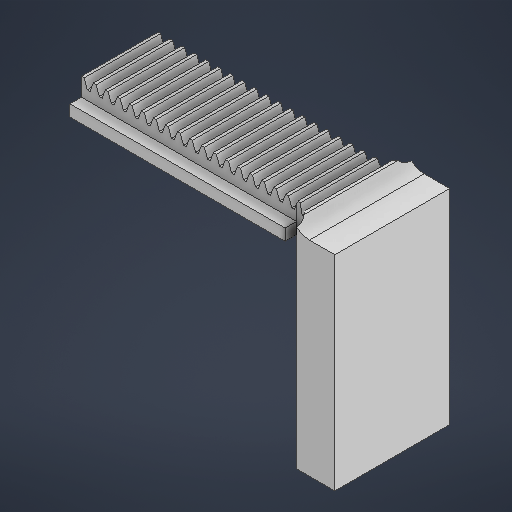
# Autodesk Inventor part: cremallera 4
Saved by Autodesk Inventor 2025.3 (Build 293356000, 356)
## iProperties
Created: 2025-10-14
Part Number: cremallera 4
Material: Genérico
Document SubType Name: Modeling
Designer: Jonathan Galarza
Density: 1 g/cm^3
Appearance: Valor por defecto
Author: Jonathan Galarza
Autodesk Inventor part; units mm, degrees
ref_plane "YZ Plane" through (0, 0, 0) normal (1, 0, 0) x (0, 1, 0)
ref_plane "XZ Plane" through (0, 0, 0) normal (0, 1, 0) x (-1, 0, 0)
ref_plane "XY Plane" through (0, 0, 0) normal (0, 0, 1) x (1, 0, 0)
sketch "Boceto1" plane through (0, 0, 0) normal (0, 0, 1) x (1, 0, 0)
  line L0 (-18.1967, 3.5798) -> (-17.4337, 3.5798)
  line L1 (-17.4337, 3.5798) -> (-16.6075, 1.3098)
  line L2 (-17.4337, 3.5798) -> (-14.4337, 3.5798) construction
  line L3 (-17.0697, 2.5798) -> (-18.5607, 2.5798) construction
  line L4 (-17.8152, 2.5798) -> (-17.8152, 2.7741) construction
  line L5 (-18.1967, 3.5798) -> (-19.023, 1.3098)
  line L6 (-15.0557, 3.5798) -> (-14.2927, 3.5798)
  line L7 (-14.2927, 3.5798) -> (-13.4665, 1.3098)
  line L8 (-13.9287, 2.5798) -> (-15.4197, 2.5798) construction
  line L9 (-14.6742, 2.5798) -> (-14.6742, 2.7741) construction
  line L10 (-15.0557, 3.5798) -> (-15.882, 1.3098)
  line L11 (-11.9147, 3.5798) -> (-11.1517, 3.5798)
  line L12 (-11.1517, 3.5798) -> (-10.3255, 1.3098)
  line L13 (-10.7877, 2.5798) -> (-12.2787, 2.5798) construction
  line L14 (-11.5332, 2.5798) -> (-11.5332, 2.7741) construction
  line L15 (-11.9147, 3.5798) -> (-12.741, 1.3098)
  line L16 (-8.7737, 3.5798) -> (-8.0107, 3.5798)
  line L17 (-8.0107, 3.5798) -> (-7.1845, 1.3098)
  line L18 (-7.6467, 2.5798) -> (-9.1377, 2.5798) construction
  line L19 (-8.3922, 2.5798) -> (-8.3922, 2.7741) construction
  line L20 (-8.7737, 3.5798) -> (-9.6, 1.3098)
  line L21 (-5.6327, 3.5798) -> (-4.8697, 3.5798)
  line L22 (-4.8697, 3.5798) -> (-4.0435, 1.3098)
  line L23 (-4.5057, 2.5798) -> (-5.9967, 2.5798) construction
  line L24 (-5.2512, 2.5798) -> (-5.2512, 2.7741) construction
  line L25 (-5.6327, 3.5798) -> (-6.459, 1.3098)
  line L26 (-2.4917, 3.5798) -> (-1.7287, 3.5798)
  line L27 (-1.7287, 3.5798) -> (-0.9025, 1.3098)
  line L28 (-1.3647, 2.5798) -> (-2.8557, 2.5798) construction
  line L29 (-2.1102, 2.5798) -> (-2.1102, 2.7741) construction
  line L30 (-2.4917, 3.5798) -> (-3.318, 1.3098)
  line L31 (0.6493, 3.5798) -> (1.4123, 3.5798)
  line L32 (1.4123, 3.5798) -> (2.2385, 1.3098)
  line L33 (1.7763, 2.5798) -> (0.2853, 2.5798) construction
  line L34 (1.0308, 2.5798) -> (1.0308, 2.7741) construction
  line L35 (0.6493, 3.5798) -> (-0.177, 1.3098)
  line L36 (3.7903, 3.5798) -> (4.5533, 3.5798)
  line L37 (4.5533, 3.5798) -> (5.3795, 1.3098)
  line L38 (4.9173, 2.5798) -> (3.4263, 2.5798) construction
  line L39 (4.1718, 2.5798) -> (4.1718, 2.7741) construction
  line L40 (3.7903, 3.5798) -> (2.964, 1.3098)
  line L41 (6.9313, 3.5798) -> (7.6943, 3.5798)
  line L42 (7.6943, 3.5798) -> (8.5205, 1.3098)
  line L43 (8.0583, 2.5798) -> (6.5673, 2.5798) construction
  line L44 (7.3128, 2.5798) -> (7.3128, 2.7741) construction
  line L45 (6.9313, 3.5798) -> (6.105, 1.3098)
  line L46 (10.0723, 3.5798) -> (10.8353, 3.5798)
  line L47 (10.8353, 3.5798) -> (11.6615, 1.3098)
  line L48 (11.1993, 2.5798) -> (9.7083, 2.5798) construction
  line L49 (10.4538, 2.5798) -> (10.4538, 2.7741) construction
  line L50 (10.0723, 3.5798) -> (9.246, 1.3098)
  line L51 (13.2133, 3.5798) -> (13.9763, 3.5798)
  line L52 (13.9763, 3.5798) -> (14.8025, 1.3098)
  line L53 (14.3403, 2.5798) -> (12.8493, 2.5798) construction
  line L54 (13.5948, 2.5798) -> (13.5948, 2.7741) construction
  line L55 (13.2133, 3.5798) -> (12.387, 1.3098)
  line L56 (16.3543, 3.5798) -> (17.1173, 3.5798)
  line L57 (17.1173, 3.5798) -> (17.9435, 1.3098)
  line L58 (17.4813, 2.5798) -> (15.9903, 2.5798) construction
  line L59 (16.7358, 2.5798) -> (16.7358, 2.7741) construction
  line L60 (16.3543, 3.5798) -> (15.528, 1.3098)
  line L61 (19.4953, 3.5798) -> (20.2583, 3.5798)
  line L62 (20.2583, 3.5798) -> (21.0845, 1.3098)
  line L63 (20.6223, 2.5798) -> (19.1313, 2.5798) construction
  line L64 (19.8768, 2.5798) -> (19.8768, 2.7741) construction
  line L65 (19.4953, 3.5798) -> (18.669, 1.3098)
  line L66 (22.6363, 3.5798) -> (23.3993, 3.5798)
  line L67 (23.3993, 3.5798) -> (24.2255, 1.3098)
  line L68 (23.7633, 2.5798) -> (22.2723, 2.5798) construction
  line L69 (23.0178, 2.5798) -> (23.0178, 2.7741) construction
  line L70 (22.6363, 3.5798) -> (21.81, 1.3098)
  line L71 (25.7773, 3.5798) -> (26.5403, 3.5798)
  line L72 (26.5403, 3.5798) -> (27.3665, 1.3098)
  line L73 (26.9043, 2.5798) -> (25.4133, 2.5798) construction
  line L74 (26.1588, 2.5798) -> (26.1588, 2.7741) construction
  line L75 (25.7773, 3.5798) -> (24.951, 1.3098)
  line L76 (28.9183, 3.5798) -> (29.6813, 3.5798)
  line L77 (29.6813, 3.5798) -> (30.5075, 1.3098)
  line L78 (30.0453, 2.5798) -> (28.5543, 2.5798) construction
  line L79 (29.2998, 2.5798) -> (29.2998, 2.7741) construction
  line L80 (28.9183, 3.5798) -> (28.092, 1.3098)
  line L81 (32.0593, 3.5798) -> (32.8223, 3.5798)
  line L82 (32.8223, 3.5798) -> (33.6485, 1.3098)
  line L83 (33.1863, 2.5798) -> (31.6953, 2.5798) construction
  line L84 (32.4408, 2.5798) -> (32.4408, 2.7741) construction
  line L85 (32.0593, 3.5798) -> (31.233, 1.3098)
  line L86 (35.2003, 3.5798) -> (35.9633, 3.5798)
  line L87 (35.9633, 3.5798) -> (36.7895, 1.3098)
  line L88 (36.3273, 2.5798) -> (34.8363, 2.5798) construction
  line L89 (35.5818, 2.5798) -> (35.5818, 2.7741) construction
  line L90 (35.2003, 3.5798) -> (34.374, 1.3098)
  line L91 (38.3413, 3.5798) -> (39.1043, 3.5798)
  line L92 (39.1043, 3.5798) -> (39.9305, 1.3098)
  line L93 (39.4683, 2.5798) -> (37.9773, 2.5798) construction
  line L94 (38.7228, 2.5798) -> (38.7228, 2.7741) construction
  line L95 (38.3413, 3.5798) -> (37.515, 1.3098)
  line L96 (41.4823, 3.5798) -> (42.2453, 3.5798)
  line L97 (42.2453, 3.5798) -> (43.0715, 1.3098)
  line L98 (42.6093, 2.5798) -> (41.1183, 2.5798) construction
  line L99 (41.8638, 2.5798) -> (41.8638, 2.7741) construction
  line L100 (41.4823, 3.5798) -> (40.656, 1.3098)
  line L101 (44.6233, 3.5798) -> (45.3863, 3.5798)
  line L102 (45.3863, 3.5798) -> (46.2125, 1.3098)
  line L103 (45.7503, 2.5798) -> (44.2593, 2.5798) construction
  line L104 (45.0048, 2.5798) -> (45.0048, 2.7741) construction
  line L105 (44.6233, 3.5798) -> (43.797, 1.3098)
  line L106 (47.7643, 3.5798) -> (48.5273, 3.5798)
  line L107 (48.5273, 3.5798) -> (49.3535, 1.3098)
  line L108 (48.8913, 2.5798) -> (47.4003, 2.5798) construction
  line L109 (48.1458, 2.5798) -> (48.1458, 2.7741) construction
  line L110 (47.7643, 3.5798) -> (46.938, 1.3098)
  line L111 (50.9053, 3.5798) -> (51.6683, 3.5798)
  line L112 (51.6683, 3.5798) -> (52.4945, 1.3098)
  line L113 (52.0323, 2.5798) -> (50.5413, 2.5798) construction
  line L114 (51.2868, 2.5798) -> (51.2868, 2.7741) construction
  line L115 (50.9053, 3.5798) -> (50.079, 1.3098)
  line L116 (54.0463, 3.5798) -> (54.8093, 3.5798)
  line L117 (54.8093, 3.5798) -> (55.6355, 1.3098)
  line L118 (55.1733, 2.5798) -> (53.6823, 2.5798) construction
  line L119 (54.4278, 2.5798) -> (54.4278, 2.7741) construction
  line L120 (54.0463, 3.5798) -> (53.22, 1.3098)
  line L121 (57.1873, 3.5798) -> (57.9503, 3.5798)
  line L122 (57.9503, 3.5798) -> (58.7765, 1.3098)
  line L123 (58.3143, 2.5798) -> (56.8233, 2.5798) construction
  line L124 (57.5688, 2.5798) -> (57.5688, 2.7741) construction
  line L125 (57.1873, 3.5798) -> (56.361, 1.3098)
  line L126 (60.3283, 3.5798) -> (61.0913, 3.5798)
  line L127 (61.0913, 3.5798) -> (61.9175, 1.3098)
  line L128 (61.4553, 2.5798) -> (59.9643, 2.5798) construction
  line L129 (60.7098, 2.5798) -> (60.7098, 2.7741) construction
  line L130 (60.3283, 3.5798) -> (59.502, 1.3098)
  line L131 (63.4693, 3.5798) -> (64.2323, 3.5798)
  line L132 (64.2323, 3.5798) -> (65.0585, 1.3098)
  line L133 (64.5963, 2.5798) -> (63.1053, 2.5798) construction
  line L134 (63.8508, 2.5798) -> (63.8508, 2.7741) construction
  line L135 (63.4693, 3.5798) -> (62.643, 1.3098)
  line L136 (66.6103, 3.5798) -> (67.3733, 3.5798)
  line L137 (67.3733, 3.5798) -> (68.1995, 1.3098)
  line L138 (67.7373, 2.5798) -> (66.2463, 2.5798) construction
  line L139 (66.9918, 2.5798) -> (66.9918, 2.7741) construction
  line L140 (66.6103, 3.5798) -> (65.784, 1.3098)
  line L141 (69.7513, 3.5798) -> (70.5143, 3.5798)
  line L142 (70.5143, 3.5798) -> (71.3405, 1.3098)
  line L143 (70.8783, 2.5798) -> (69.3873, 2.5798) construction
  line L144 (70.1328, 2.5798) -> (70.1328, 2.7741) construction
  line L145 (69.7513, 3.5798) -> (68.925, 1.3098)
  line L146 (72.8923, 3.5798) -> (73.6553, 3.5798)
  line L147 (73.6553, 3.5798) -> (74.4815, 1.3098)
  line L148 (74.0193, 2.5798) -> (72.5283, 2.5798) construction
  line L149 (73.2738, 2.5798) -> (73.2738, 2.7741) construction
  line L150 (72.8923, 3.5798) -> (72.066, 1.3098)
  line L151 (-19.023, 1.3098) -> (74.4815, 1.3098)
  line L152 (74.4815, 1.3098) -> (74.4815, -4.1423)
  line L153 (74.4815, -4.1423) -> (-19.023, -4.1423)
  line L154 (-19.023, -4.1423) -> (-19.023, 1.3098)
  point P0 (0, 0)
  point P1 (-16.4076, 0.7607)
  point P2 (-19.2228, 0.7607)
  dimension "d3" = 3
  dimension "d4" = 70
  dimension "d5" = 1.491
  dimension "d8" = 3.141
  constraints: 308 end point, 30 point on line, 3 horizontal, 2 symmetric about line, 2 vertical, 1 midpoint, 1 parallel, 380 other
  measures "d3" distance of L0.end point (-16.408, 0.761)
  measures "d4" angle of L1 L2
  measures "d5" distance of L3.start L3.end
  measures "d8" distance of L0.start L6.start
extrude "Extrusión1" add sketch "Boceto1" along normal blind 20
sketch "Boceto3" plane through (74.4815, -4.1423, 0) normal (1, 0, 0) x (0, 0, -1)
  line L0 (0, 7.7221) -> (-20, 7.7221) projected
  line L1 (-25, 5.4521) -> (-25, -47.9849)
  line L2 (-25, -47.9849) -> (5, -47.9849)
  line L3 (0, 5.4521) -> (-20, 5.4521) projected
  line L4 (-10, 5.4521) -> (-25, 5.4521)
  line L5 (-10, 5.4521) -> (5, 5.4521)
  line L6 (5, 5.4521) -> (5, -47.9849)
  point P0 (0, 4.1423)
  dimension "d18" = 53.437
  dimension "d19" = 30
  dimension "d20" = 15
  constraints: 10 end point, 3 perpendicular, 1 midpoint, 1 point on line
  measures "d18" distance of L1.start L1.end
  measures "d19" distance of L1.end L2.end
  measures "d20" distance of L4.start L5.end
extrude "Extrusión3" add sketch "Boceto3" along normal blind 10
sketch "Boceto5" plane through (-19.023, -4.1423, 0) normal (-1, 0, 0) x (0, 0, 1)
  line L0 (-17.8231, 19.901) -> (36.2656, 19.901)
  line L1 (36.2656, 19.901) -> (36.2656, -7.4874)
  line L2 (36.2656, -7.4874) -> (-17.8231, -7.4874)
  line L3 (-17.8231, -7.4874) -> (-17.8231, 19.901)
  point P0 (0, 4.1423)
  constraints: 8 end point, 2 parallel, 1 horizontal, 1 perpendicular
extrude "Extrusión5" cut sketch "Boceto5" against normal blind 32.3
sketch "Boceto6" plane through (13.277, -4.1423, 0) normal (-1, 0, 0) x (0, 0, 1)
  line L0 (20, 0) -> (0, 0) projected
  line L1 (20, 7.7221) -> (20, 0) projected
  line L2 (0, 7.7221) -> (20, 7.7221) projected
  line L3 (0, 0) -> (0, 7.7221) projected
  line L4 (0, 0) -> (-3, 0)
  line L5 (-3, 0) -> (-3, 3)
  line L6 (-3, 3) -> (0, 3)
  line L7 (0, 3) -> (0, 0)
  line L8 (20, 0) -> (23, 0)
  line L9 (23, 0) -> (23, 3)
  line L10 (23, 3) -> (20, 3)
  line L11 (20, 3) -> (20, 0)
  point P0 (0, 4.1423)
  dimension "d35" = 3
  dimension "d36" = 3
  dimension "d37" = 3
  dimension "d38" = 3
  constraints: 16 end point, 4 parallel, 2 horizontal, 2 perpendicular
  measures "d35" distance of L5.end L6.end
  measures "d36" distance of L4.end L5.end
  measures "d37" distance of L10.end L9.end
  measures "d38" distance of L9.end L8.end
extrude "Extrusión6" add sketch "Boceto6" against normal blind 56.2045 contours L1 L10 L9 L8 | L4 L5 L6 L3
fillet "Empalme3" radius 5 3 edges at (74.4815, 1.3098, 10) (74.4815, -1.4163, 20) (74.4815, -1.4163, 0)
fillet "Empalme4" radius 3 1 edges at (74.4815, -4.1423, 10)
